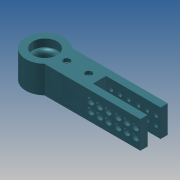
# Autodesk Inventor part: driven arm 2_1
Saved by Autodesk Inventor 2013 (Build 170138000, 138)
## iProperties
Created: 2017-03-30
Part Number: driven arm 2_1
Material: Generic
Document SubType Name: Modeling
Designer: employee
Density: 1 g/cm^3
Author: employee
Autodesk Inventor part; units mm, degrees
ref_plane "YZ Plane" through (0, 0, 0) normal (1, 0, 0) x (0, 1, 0)
ref_plane "XZ Plane" through (0, 0, 0) normal (0, 1, 0) x (-1, 0, 0)
ref_plane "XY Plane" through (0, 0, 0) normal (0, 0, 1) x (1, 0, 0)
sketch "Sketch1" plane through (0, 0, 0) normal (0, 0, 1) x (1, 0, 0)
  line L0 (0, 12.6) -> (150, 12.6)
  arc A0 (150, -12.6) -> (150, 12.6) centre (150, 0) ccw
  line L1 (150, -12.6) -> (0, -12.6)
  arc A1 (0, 12.6) -> (0, -12.6) centre (0, 0) ccw
  circle A2 centre (0, 0) radius 7.5
  circle A3 centre (150, 0) radius 4.25
  dimension "d0" = 150
  dimension "d2" = 12.6
  dimension "d3" = 15
  dimension "d4" = 8.5
  constraints: 4 centre point, 4 end point, 4 point on circle, 4 tangent, 3 coincident, 1 horizontal, 1 parallel
  measures "d0" distance of L0.start L0.end
  measures "d2" radius of A1
  measures "d3" diameter of A2
  measures "d4" diameter of A3
extrude "Extrusion1" add sketch "Sketch1" along normal blind 25
sketch "Sketch2" plane through (0, 0, 25) normal (0, 0, 1) x (1, 0, 0)
  circle A0 centre (0, 0) radius 7.5 projected
  arc A1 (0, 12.6) -> (0, -12.6) centre (0, 0) ccw projected
  circle A2 centre (0, 0) radius 11
  dimension "d7" = 22
  constraints: 1 centre point, 1 coincident
  measures "d7" diameter of A2
extrude "Extrusion2" cut sketch "Sketch2" against normal blind 7
sketch "Sketch4" plane through (0, 0, 25) normal (0, 0, 1) x (1, 0, 0)
  circle A0 centre (0, 0) radius 11 projected
  circle A1 centre (20, 0) radius 1.75
  circle A2 centre (40, 0) radius 1.75
  dimension "d16" = 20
  dimension "d17" = 40
  dimension "d23" = 3.5
  constraints: 2 centre point, 2 horizontal alignment, 1 equal radius
  measures "d16" distance of A1.centre A0.centre
  measures "d17" distance of A2.centre A0.centre
  measures "d23" diameter of A1
extrude "Extrusion3" cut sketch "Sketch4" against normal through all contours A1 | A2
sketch "Sketch5" plane through (0, 0, 25) normal (0, 0, 1) x (1, 0, 0)
  circle A0 centre (20, 0) radius 1.75 projected
  circle A1 centre (40, 0) radius 1.75 projected
  circle A2 centre (40, 0) radius 3
  circle A3 centre (20, 0) radius 3
  dimension "d28" = 6
  constraints: 2 centre point, 2 coincident, 1 equal radius
  measures "d28" diameter of A3
extrude "Extrusion4" cut sketch "Sketch5" against normal blind 3
sketch "Sketch6" plane through (0, 0, 25) normal (0, 0, 1) x (1, 0, 0)
  line L0 (150, 12.6) -> (0, 12.6) projected
  arc A0 (0, 12.6) -> (0, -12.6) centre (0, 0) ccw projected
  line L1 (0, -12.6) -> (150, -12.6) projected
  arc A1 (12.1445, 12.6) -> (12.1445, -12.6) centre (0, 0) ccw
  dimension "d24" = 35
  constraints: 2 point on circle, 2 point on line, 1 centre point, 1 coincident
  measures "d24" diameter of A1
extrude "Extrusion5" add sketch "Sketch6" against normal up to surface (25 mm away)
sketch "Sketch7" plane through (0, 0, 25) normal (0, 0, 1) x (1, 0, 0)
  circle A0 centre (150, 0) radius 4.25 projected
  arc A1 (150, -12.6) -> (150, 12.6) centre (150, 0) ccw projected
  circle A2 centre (150, 0) radius 7
  dimension "d30" = 14
  constraints: 1 centre point, 1 coincident
  measures "d30" diameter of A2
extrude "Extrusion6" cut sketch "Sketch7" against normal blind 8
fillet "Fillet1" radius 3.5 1 edges at (-7.5, 0, 18)
sketch "Sketch8" plane through (0, 0, 25) normal (0, 0, 1) x (1, 0, 0)
  circle A0 centre (150, 0) radius 7 projected
  line L0 (150, 12.6) -> (12.1445, 12.6) projected
  line L1 (12.1445, -12.6) -> (150, -12.6) projected
  arc A1 (150, -12.6) -> (150, 12.6) centre (150, 0) ccw projected
  line L2 (100, 12.6) -> (100, 6)
  line L3 (100, 6) -> (50, 6)
  line L4 (50, 6) -> (50, -6)
  line L5 (50, -6) -> (100, -6)
  line L6 (100, -6) -> (100, -12.6)
  point P0 (50, 0)
  dimension "d35" = 12
  dimension "d37" = 50
  dimension "d38" = 50
  constraints: 10 end point, 3 parallel, 3 perpendicular, 2 point on line, 1 horizontal alignment, 1 midpoint
  measures "d35" distance of L3.end L4.end
  measures "d37" distance of L2.end L3.end
  measures "d38" distance from line of L2 A0.centre
extrude "Extrusion7" cut sketch "Sketch8" against normal through all contours A0 | A1 L1 L6 L5 L4 L3 L2 L0
sketch "Sketch9" plane through (12.1445, -12.6, 0) normal (0, -1, 0) x (1, 0, 0)
  line L0 (87.8555, 0) -> (87.8555, 25) projected
  line L1 (83.3555, 8.5) -> (75.3555, 8.5)
  line L2 (75.3555, 8.5) -> (75.3555, 16.5)
  line L3 (75.3555, 16.5) -> (83.3555, 16.5)
  line L4 (83.3555, 16.5) -> (83.3555, 8.5)
  line L5 (75.3555, 16.5) -> (67.3555, 16.5)
  line L6 (67.3555, 16.5) -> (67.3555, 8.5)
  line L7 (67.3555, 8.5) -> (75.3555, 8.5)
  line L8 (75.3555, 8.5) -> (75.3555, 16.5)
  circle A0 centre (67.3555, 16.5) radius 1.75
  point P0 (-12.1445, 0)
  point P1 (75.3555, 12.5)
  point P2 (87.8555, 12.5)
  dimension "d41" = 12.5
  dimension "d42" = 8
  dimension "d43" = 3.5
  constraints: 16 end point, 4 parallel, 2 equal length, 2 horizontal, 2 midpoint, 2 perpendicular, 1 centre point, 1 coincident, 1 horizontal alignment, 1 point on line
  measures "d41" distance from line of L2.end L0
  measures "d42" distance of L2.end L3.end
  measures "d43" diameter of A0
extrude "Extrusion8" cut sketch "Sketch9" against normal through all contours A0 L6 L5 | L5 L6 A0
sketch "Sketch10" plane through (12.1445, -12.6, 0) normal (0, -1, 0) x (1, 0, 0)
  circle A0 centre (67.3555, 16.5) radius 1.75 projected
  circle A1 centre (67.3555, 16.5) radius 3
  point P0 (-12.1445, 0)
  dimension "d46" = 6
  constraints: 1 centre point, 1 coincident
  measures "d46" diameter of A1
extrude "Extrusion9" cut sketch "Sketch10" against normal blind 3
sketch "Sketch11" plane through (12.1445, 12.6, 25) normal (0, 1, 0) x (1, 0, 0)
  circle A0 centre (67.3555, 8.5) radius 1.75 projected
  line L0 (64.18, 8.5) -> (65.7677, 11.25)
  line L1 (65.7677, 11.25) -> (68.9432, 11.25)
  line L2 (68.9432, 11.25) -> (70.5309, 8.5)
  line L3 (70.5309, 8.5) -> (68.9432, 5.75)
  line L4 (68.9432, 5.75) -> (65.7677, 5.75)
  line L5 (65.7677, 5.75) -> (64.18, 8.5)
  point P0 (-12.1445, 25)
  dimension "d50" = 5.5
  constraints: 12 end point, 1 coincident, 1 horizontal, 13 other
  measures "d50" distance between parallel lines of L4 L1
extrude "Extrusion10" cut sketch "Sketch11" against normal blind 4
pattern_linear "Rectangular Pattern1" count 3 spacing 8 along (1, 0, 0) count 2 spacing 8 along (0, 0, -1) of "Extrusion10", "Extrusion9", "Extrusion8"
pattern_linear "Rectangular Pattern2" count 2 spacing 25 along (-1, 0, 0) of "Extrusion10", "Extrusion9", "Extrusion8", "Rectangular Pattern1"
body "Solid1"
